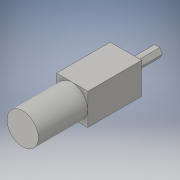
# Autodesk Inventor part: Bag elevator Motor
Saved by Autodesk Inventor 2016 SP2 (Build 200236200, 236)
## iProperties
Created: 2018-02-02
Part Number: Bag elevator Motor
Material: Generic
Document SubType Name: Modeling
Designer: CAD
Density: 1 g/cm^3
Appearance: Default
Author: CAD
Autodesk Inventor part; units mm, degrees
ref_plane "YZ Plane" through (0, 0, 0) normal (1, 0, 0) x (0, 1, 0)
ref_plane "XZ Plane" through (0, 0, 0) normal (0, 1, 0) x (-1, 0, 0)
ref_plane "XY Plane" through (0, 0, 0) normal (0, 0, 1) x (1, 0, 0)
sketch "Sketch1" plane through (0, 0, 0) normal (0, 0, 1) x (1, 0, 0)
  line L0 (0, 0) -> (0, 44.45)
  line L1 (0, 0) -> (44.45, 0)
  line L2 (44.45, 0) -> (44.45, 44.45)
  line L3 (44.45, 44.45) -> (0, 44.45)
  dimension "d1" = 44.45
  dimension "d2" = 44.45
  constraints: 8 end point, 2 perpendicular, 1 horizontal, 1 vertical
  measures "d1" distance of L0.start L0.end
  measures "d2" distance of L0.start L1.end
extrude "Extrusion1" add sketch "Sketch1" along normal blind 76.2
sketch "Sketch2" plane through (0, 0, 76.2) normal (0, 0, 1) x (1, 0, 0)
  circle A0 centre (22.225, 22.225) radius 22.225
  line L0 (44.45, 44.45) -> (0, 44.45) projected
  line L1 (44.45, 0) -> (44.45, 44.45) projected
  point P0 (0, 0)
  dimension "d5" = 44.45
  dimension "d6" = 22.225
  dimension "d7" = 22.225
  constraints: 1 centre point
  measures "d5" diameter of A0
  measures "d6" distance from line of L0 A0.centre
  measures "d7" distance from line of L1 A0.centre
extrude "Extrusion2" add sketch "Sketch2" along normal blind 69.85 contours A0
sketch "Sketch3" plane through (0, 0, 0) normal (0, 0, -1) x (-1, 0, 0)
  line L0 (-18.5588, 15.875) -> (-25.8912, 15.875)
  line L1 (-25.8912, 15.875) -> (-29.5573, 22.225)
  line L2 (-29.5573, 22.225) -> (-25.8912, 28.575)
  line L3 (-25.8912, 28.575) -> (-18.5588, 28.575)
  line L4 (-18.5588, 28.575) -> (-14.8927, 22.225)
  line L5 (-14.8927, 22.225) -> (-18.5588, 15.875)
  line L6 (-44.45, 0) -> (0, 0) projected
  line L7 (0, 0) -> (0, 44.45) projected
  point P0 (-22.225, 22.225)
  dimension "d10" = 12.7
  dimension "d11" = 22.225
  dimension "d12" = 22.225
  constraints: 12 end point, 1 horizontal, 13 other
  measures "d10" distance between parallel lines of L2 L5
  measures "d11" distance from line of L6 point (-22.225, 22.225)
  measures "d12" distance from line of L7 point (-22.225, 22.225)
extrude "Extrusion3" add sketch "Sketch3" along normal blind 44.45
body "Solid1"
